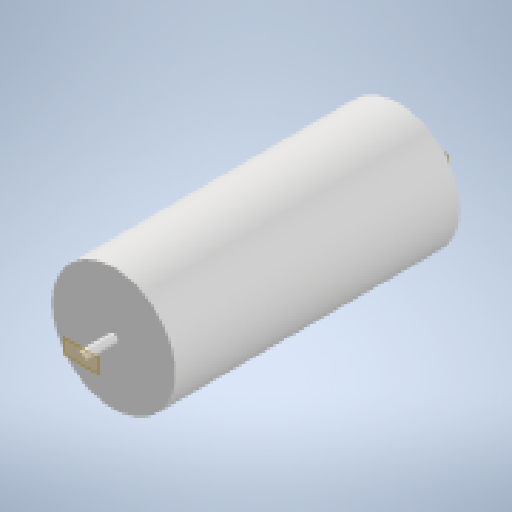
# Autodesk Inventor part: LONGI_BRUSH
Saved by Autodesk Inventor 2024 (Build 280153000, 153)
## iProperties
Created: 2024-04-16
Part Number: LONGI_BRUSH
Material: Generic
Document SubType Name: Modeling
Designer: teeta
Density: 1 g/cm^3
Appearance: Default
Author: teeta
Autodesk Inventor part; units mm, degrees
ref_plane "YZ Plane" through (0, 0, 0) normal (1, 0, 0) x (0, 1, 0)
ref_plane "XZ Plane" through (0, 0, 0) normal (0, 1, 0) x (-1, 0, 0)
ref_plane "XY Plane" through (0, 0, 0) normal (0, 0, 1) x (1, 0, 0)
ref_plane "Work Plane1" through (0, 0, -19.5) normal (0, 0, 1) x (1, 0, 0)
sketch "Sketch1" plane through (0, 0, -19.5) normal (0, 0, 1) x (1, 0, 0)
  circle A0 centre (37.4246, 12.4618) radius 10
  point P0 (0, 0)
  dimension "d0" = 20
  constraints: 1 centre point
  measures "d0" diameter of A0
ref_plane "Work Plane2" through (74.8493, 0, -818.6) normal (0, 0, -1) x (-1, 0, 0)
extrude "Extrusion1" add sketch "Sketch1" against normal up to surface (799.1 mm away)
ref_plane "Work Plane3" through (0, 0, -419.05) normal (0, 0, 1) x (1, 0, 0)
sketch "Sketch2" plane through (0, 0, -419.05) normal (0, 0, 1) x (1, 0, 0)
  circle A0 centre (37.4246, 12.4618) radius 10 projected
  circle A1 centre (37.4246, 12.4618) radius 140
  point P0 (0, 0)
  dimension "d3" = 280
  constraints: 1 centre point, 1 coincident
  measures "d3" diameter of A1
extrude "Extrusion2" add sketch "Sketch2" along normal mid plane 650
body "Solid1"
